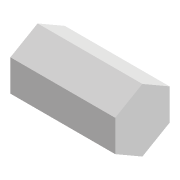
# Autodesk Inventor part: 关节2
Saved by Autodesk Inventor 2022 (Build 260153000, 153)
## iProperties
Created: 2023-03-20
Part Number: 关节2
Material: 常规
Document SubType Name: Modeling
Designer: Lzy18
Density: 1 g/cm^3
Appearance: 默认
Author: Lzy18
Autodesk Inventor part; units mm, degrees
ref_plane "YZ Plane" through (0, 0, 0) normal (1, 0, 0) x (0, 1, 0)
ref_plane "XZ Plane" through (0, 0, 0) normal (0, 1, 0) x (-1, 0, 0)
ref_plane "XY Plane" through (0, 0, 0) normal (0, 0, 1) x (1, 0, 0)
sketch "草图1" plane through (0, 0, 0) normal (1, 0, 0) x (0, 1, 0)
  line L0 (3.6213, 2.1213) -> (1.5, 0)
  line L1 (1.5, 0) -> (-1.5, 0)
  line L2 (-1.5, 0) -> (-3.6213, 2.1213)
  line L3 (-3.6213, 2.1213) -> (-3.6213, 5.1213)
  line L4 (-3.6213, 5.1213) -> (-1.5, 7.2426)
  line L5 (-1.5, 7.2426) -> (1.5, 7.2426)
  line L6 (1.5, 7.2426) -> (3.6213, 5.1213)
  line L7 (3.6213, 5.1213) -> (3.6213, 2.1213)
  line L8 (1.608, 0) -> (-1.392, 0) projected
  line L9 (0, 0) -> (0, 9.8594)
  point P0 (0, 3.6213)
  dimension "d0" = 3
  constraints: 18 end point, 2 collinear, 1 point on line, 1 vertical, 17 other
  measures "d0" distance of L1.end L0.end
extrude "拉伸1" add sketch "草图1" along normal mid plane 10
sketch "草图2" plane through (-5, 0, 0) normal (-1, 0, 0) x (0, 0, 1)
  line L0 (2.1213, -3.6213) -> (5.1213, -3.6213) projected
  line L1 (5.1213, -3.6213) -> (7.2426, -1.5) projected
  line L2 (7.2426, -1.5) -> (7.2426, 1.5) projected
  line L3 (7.2426, 1.5) -> (5.1213, 3.6213) projected
  line L4 (5.1213, 3.6213) -> (2.1213, 3.6213) projected
  line L5 (2.1213, 3.6213) -> (0, 1.5) projected
  line L6 (0, 1.5) -> (0, -1.5) projected
  line L7 (0, -1.5) -> (2.1213, -3.6213) projected
  circle A0 centre (3.6213, 0) radius 1.5
  point P0 (0, 0)
  dimension "d3" = 3
  constraints: 1 centre point
  measures "d3" diameter of A0
hole "孔1" at (-5, 0, 3.6213) direction (1, 0, 0) diameter 3 end through all
